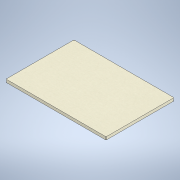
# Autodesk Inventor part: FactionMats_All
Saved by Autodesk Inventor 2021 (Build 250183000, 183)
## iProperties
Created: 2023-03-16
Part Number: FactionMats_All
Material: Paper
Document SubType Name: Modeling
Designer: Bradley
Density: 0.93 g/cm^3
Appearance: Cardboard - Chipboard
Author: Bradley
Autodesk Inventor part; units mm, degrees
ref_plane "YZ Plane" through (0, 0, 0) normal (1, 0, 0) x (0, 1, 0)
ref_plane "XZ Plane" through (0, 0, 0) normal (0, 1, 0) x (-1, 0, 0)
ref_plane "XY Plane" through (0, 0, 0) normal (0, 0, 1) x (1, 0, 0)
sketch "Sketch1" plane through (0, 0, 0) normal (0, 1, 0) x (-1, 0, 0)
  line L0 (138, 95) -> (-138, 95)
  line L1 (-140, 93) -> (-140, -93)
  line L2 (-138, -95) -> (138, -95)
  line L3 (140, -93) -> (140, 93)
  line L4 (140, 95) -> (-140, -95) construction
  line L5 (-140, 95) -> (140, -95) construction
  arc A0 (138, -95) -> (140, -93) centre (138, -93) ccw
  arc A1 (140, 93) -> (138, 95) centre (138, 93) ccw
  arc A2 (-138, 95) -> (-140, 93) centre (-138, 93) ccw
  arc A3 (-140, -93) -> (-138, -95) centre (-138, -93) ccw
  point P0 (0, 0)
  dimension "d0" = 280
  dimension "d1" = 190
  dimension "d2" = 2
  constraints: 12 end point, 8 point on circle, 8 point on line, 8 tangent, 4 centre point, 3 equal radius, 2 midpoint, 2 parallel, 1 horizontal, 1 perpendicular
  measures "d0" distance of L5.end L4.end
  measures "d1" distance of L4.end L5.start
  measures "d2" radius of A0
extrude "Extrusion1" add sketch "Sketch1" along normal mid plane 8
body "Solid1"
